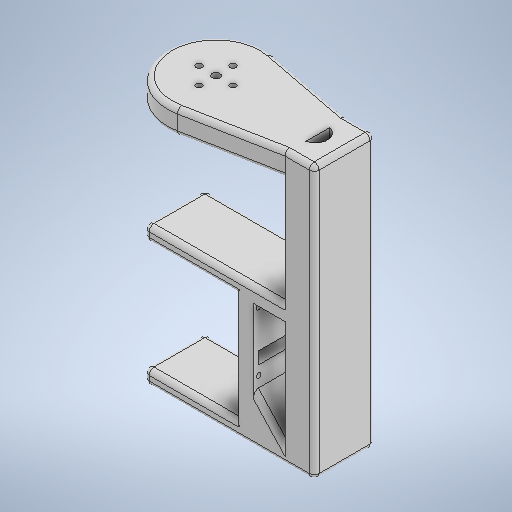
# Autodesk Inventor part: wahacz
Saved by Autodesk Inventor 2025.3 (Build 293356000, 356)
## iProperties
Created: 2026-03-17
Part Number: wahacz
Material: Generic
Document SubType Name: Modeling
Designer: ksawe
Density: 1 g/cm^3
Appearance: Default
Author: ksawe
Autodesk Inventor part; units mm, degrees
ref_plane "YZ Plane" through (0, 0, 0) normal (1, 0, 0) x (0, 1, 0)
ref_plane "XZ Plane" through (0, 0, 0) normal (0, 1, 0) x (-1, 0, 0)
ref_plane "XY Plane" through (0, 0, 0) normal (0, 0, 1) x (1, 0, 0)
sketch "Sketch1" plane through (0, 0, 0) normal (0, 0, 1) x (1, 0, 0)
  line L0 (5, -71.22) -> (5, -26)
  line L1 (5, -26) -> (-34, -26)
  line L2 (-34, -20) -> (24, -20)
  line L3 (-34, -20) -> (-34, -26)
  line L4 (-34, -20) -> (24, -20)
  line L5 (24, -20) -> (-34, -20)
  line L6 (36, 35) -> (24, 35)
  line L7 (24, 35) -> (24, -20)
  line L8 (11, -26) -> (11, -57.22)
  line L9 (24, -71.22) -> (24, -26)
  line L10 (24, -26) -> (11, -26)
  line L11 (-34, -71.22) -> (-34, -77.22)
  line L12 (-34, -77.22) -> (36, -77.22)
  line L13 (36, 35) -> (36, -77.22)
  line L14 (5, -71.22) -> (-34, -71.22)
  line L15 (11, -57.22) -> (24, -71.22)
  point P0 (10, -14)
  dimension "d121" = 12
  dimension "d257" = 6
  dimension "d259" = 58
  dimension "d260" = 39
  dimension "d261" = 6
  dimension "d263" = 6
  dimension "d281" = 70
  dimension "d283" = 55
  dimension "d285" = 112.22
  dimension "d307" = 106.22
  dimension "d319" = 14
  dimension "d321" = 31.22
  constraints: 32 end point, 4 vertical, 4 vertical alignment, 2 horizontal alignment, 1 horizontal, 1 parallel, 1 perpendicular
  measures "d121" distance of L6.start L6.end
  measures "d257" distance of L2.start L1.end
  measures "d259" distance of L2.start L2.end
  measures "d260" distance from line of L1.end L0
  measures "d261" distance between parallel lines of L8 L0
  measures "d263" distance of L11.start L11.end
  measures "d281" distance of L11.end L12.end
  measures "d283" distance between parallel lines of L2 L6
  measures "d285" distance of L6.start L12.end
  measures "d307" distance from line of L9.start L6
  measures "d319" distance from line of L14 L8.end
  measures "d321" distance of L8.start L8.end
extrude "Extrusion1" add sketch "Sketch1" along normal blind 25
sketch "Sketch3" plane through (24, 35, 0) normal (0, 1, 0) x (1, 0, 0)
  arc A0 (-37.1774, 7.141) -> (-37.1774, -32.141) centre (-40.95, -12.5) ccw
  line L0 (0, 0) -> (0, -25) projected
  line L1 (12, 0) -> (0, 0) projected
  line L2 (0, 0) -> (-37.1774, 7.141)
  line L3 (0, -25) -> (-37.1774, -32.141)
  line L4 (12, 0) -> (12, -25) projected
  point P0 (-24, 0)
  dimension "d137" = 40
  dimension "d231" = 52.95
  dimension "d233" = 12.5
  constraints: 4 end point, 2 point on circle, 2 tangent, 1 centre point
  measures "d137" diameter of A0
  measures "d231" distance from line of L4 A0.centre
  measures "d233" vertical distance of point (-24, 0) A0.centre
extrude "Extrusion3" add sketch "Sketch3" against normal blind 10
sketch "Sketch13" plane through (36, 35, 25) normal (0, 1, 0) x (1, 0, 0)
  arc A0 (-49.1774, 32.141) -> (-49.1774, -7.141) centre (-52.95, 12.5) ccw projected
  circle A1 centre (-52.95, 12.5) radius 1.6
  circle A2 centre (-52.95, 19.5) radius 1.25
  circle A3 centre (-59.95, 12.5) radius 1.25
  circle A4 centre (-52.95, 5.5) radius 1.25
  circle A5 centre (-45.95, 12.5) radius 1.25
  point P0 (-36, 25)
  dimension "d218" = 3.2
  dimension "d219" = 2.5
  dimension "d222" = 360
  dimension "d224" = 7
  dimension "d225" = 7
  constraints: 5 centre point, 1 coincident, 9 other
  measures "d218" diameter of A1
  measures "d219" diameter of A2
  measures "d224" horizontal distance of A2.centre A5.centre
  measures "d225" distance of A5.centre A0.centre
extrude "Extrusion6" cut sketch "Sketch13" against normal blind 10
fillet "Fillet1" radius 2 17 edges at (-5, -20, 25) (-5, -20, 0) (-34, -20, 12.5) (-34, -26, 12.5) (-14.5, -26, 0) (-14.5, -26, 25) (-36.95, 35, 12.5) (5.4113, 35, -3.5705) (5.4113, 35, 28.5705) (-36.95, 25, 12.5) (5.4113, 25, -3.5705) (5.4113, 25, 28.5705) (36, -77.22, 12.5) (36, 35, 12.5) (30, 35, 25) (30, 35, 0) (-34, -71.22, 12.5)
sketch "Sketch14" plane through (23.8097, 35, 2) normal (0, 1, 0) x (1, 0, 0)
  line L0 (0.1903, -20.9634) -> (0.1903, -0.0366) projected
  circle A0 centre (0.1903, -10.5) radius 5
  point P0 (-23.8097, 2)
  point P1 (0.1903, -5.5)
  point P2 (0.1903, -15.5)
  dimension "d275" = 10
  constraints: 1 centre point, 1 midpoint
  measures "d275" diameter of A0
sketch "Sketch16" plane through (11, -71.22, 0) normal (1, 0, 0) x (0, 0, -1)
  line L0 (0, 45.22) -> (-25, 45.22) projected
  line L1 (-12.5, 45.22) -> (-12.5, -2)
  line L2 (0, -2) -> (-25, -2) projected
  circle A0 centre (-22.89, 42.86) radius 1
  circle A1 centre (-22.89, 18.41) radius 1
  line L3 (-22.89, 27.22) -> (-2.11, 27.22)
  line L4 (-2.11, 27.22) -> (-2.11, 22.22)
  line L5 (-2.11, 22.22) -> (-22.89, 22.22)
  line L6 (-22.89, 22.22) -> (-22.89, 27.22)
  line L7 (-25, 14) -> (-25, 45.22) projected
  circle A2 centre (-2.11, 42.86) radius 1
  circle A3 centre (-2.11, 18.41) radius 1
  line L8 (0, 0) -> (-25, 0) projected
  point P0 (0, 71.22)
  point P1 (-22.89, 24.72)
  point P2 (-2.11, 24.72)
  dimension "d264" = 2
  dimension "d265" = 2
  dimension "d266" = 24.45
  dimension "d268" = 2.11
  dimension "d269" = 18
  dimension "d270" = 23
  dimension "d280" = 18.41
  constraints: 10 end point, 4 centre point, 4 midpoint, 3 vertical alignment, 2 parallel, 2 symmetric about line, 1 horizontal, 1 perpendicular, 2 other
  measures "d264" diameter of A0
  measures "d265" diameter of A1
  measures "d266" distance of A1.centre A0.centre
  measures "d268" distance from line of L7 A1.centre
  measures "d269" distance between parallel lines of L0 L3
  measures "d270" distance between parallel lines of L0 L5
  measures "d280" distance from line of L8 A1.centre
extrude "Extrusion7" cut sketch "Sketch16" against normal through all
extrude "Extrusion8" cut sketch "Sketch14" against normal blind 65 contours L0 A0 picked at (1.4934, -9.4609)
sketch "Sketch19" plane through (-32, -20, 2) normal (0, 1, 0) x (1, 0, 0)
  line L0 (56, 0) -> (56, -5.5) projected
  line L1 (56, -5.5) -> (57, -5.5)
  line L2 (57, -5.5) -> (57, -15.5)
  line L3 (57, -15.5) -> (56, -15.5)
  line L4 (56, -15.5) -> (56, -5.5)
  point P0 (32, 2)
  dimension "d314" = 1
  dimension "d315" = 10
  constraints: 8 end point, 2 parallel, 1 horizontal, 1 perpendicular
  measures "d314" distance between parallel lines of L4 L2
  measures "d315" distance of L1.end L2.end
extrude "Extrusion11" add sketch "Sketch19" along normal up to surface (55 mm away)
fillet "Fillet2" radius 2 23 edges at (35.4142, -76.6342, 25) (36, -21.11, 25) (35.4142, 34.4142, 24.4142) (0, -77.22, 25) (35.4142, -76.6342, 0) (36, -21.11, 0) (35.4142, 34.4142, 0.5858) (0, -77.22, 0) (17.5, -64.22, 25) (17.5, -64.22, 0) (-33.4142, -71.8058, 25) (-13.5, -71.22, 25) (-34, -75.22, 25) (-33.4142, -71.8058, 0) (-13.5, -71.22, 0) (-34, -75.22, 0) (-34, -77.22, 12.5) (-33.4142, -25.4142, 24.4142) (-33.4142, -20.5858, 24.4142) (-34, -23, 25) (-33.4142, -25.4142, 0.5858) (-33.4142, -20.5858, 0.5858) (-34, -23, 0)
body "Solid1"
